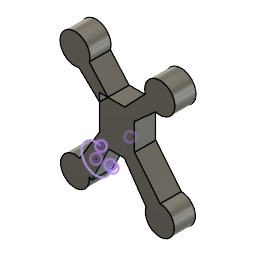
drona (Autodesk Fusion 360 design; units mm, degrees)
part number: 2026-07-06-18-59-21-464
Autodesk Fusion 360 part; units mm, degrees
sketch "Sketch1" plane through (0, 0, 0) normal (0, 0, 1) x (1, 0, 0)
  line L0 (-84.5803, 129.3728) -> (80, 129.3728)
  line L1 (80, 129.3728) -> (80, -80)
  line L2 (80, -80) -> (-84.5803, -80)
  line L3 (-84.5803, -80) -> (-84.5803, 129.3728)
  line L4 (-150, 250) -> (-200, 200)
  line L5 (-200, 200) -> (-84.5803, 90.0801)
  line L6 (-44.3949, 129.3728) -> (-84.5803, 90.0801)
  line L7 (-150, 250) -> (-44.3949, 129.3728)
  constraint horizontal L0
  constraint vertical L1
  constraint horizontal L2
  constraint vertical L3
  constraint coincident L3 L5.end
  constraint coincident L0 L6.start
sketch "Sketch2" plane through (0, 0, 0) normal (0, 0, 1) x (1, 0, 0)
sketch "Sketch3" plane through (0, 0, 0) normal (0, 0, 1) x (1, 0, 0)
sketch "Sketch4" plane through (0, 0, 0) normal (0, 0, 1) x (1, 0, 0)
  line L0 (36.1891, 130.6348) -> (78.7424, 91.729)
  line L1 (200, 200) -> (78.7424, 91.729)
  line L2 (200, 200) -> (150, 250)
  line L3 (150, 250) -> (36.1891, 130.6348)
sketch "Sketch5" plane through (0, 0, 0) normal (0, 0, 1) x (1, 0, 0)
  line L0 (-82.675, -29.7873) -> (-38.9059, -78.4196)
  line L1 (-38.9059, -78.4196) -> (-120.6501, -247.4815)
  line L2 (-120.6501, -247.4815) -> (-189.9512, -207.3598)
  line L3 (-189.9512, -207.3598) -> (-82.675, -29.7873)
sketch "Sketch6" plane through (0, 0, 0) normal (0, 0, 1) x (1, 0, 0)
  line L0 (31.611, -78.4196) -> (81.4591, -32.2189)
  line L1 (81.4591, -32.2189) -> (213.6971, -196.4176)
  line L2 (213.6971, -196.4176) -> (150, -250)
  line L3 (31.611, -78.4196) -> (150, -250)
sketch "Sketch7" plane through (0, 0, 0) normal (0, 0, 1) x (1, 0, 0)
  circle A0 centre (200, 250) radius 71.2765
  circle A1 centre (200, -250) radius 68.2747
  circle A2 centre (-200, 250) radius 70.7107
  circle A3 centre (-200, -250) radius 67.9593
extrude "Extrude1" add sketch "Sketch1" sketch "Sketch7" sketch "Sketch4" sketch "Sketch6" sketch "Sketch5" along normal blind 100 contours L0 L3 L4 L5 L7 | L0 L1 L2 L3 L6 of sketch 2 of sketch 3 of sketch 4 of sketch 5 makes body 1
surface "SurfacePatch1" add patch along 3 edges at (-64.4876, 129.3728, 0) (-64.4876, 109.7265, 0) (-84.5803, 109.7265, 0) separate body on bodies 1 makes body 2
sketch "Sketch8" plane through (0, 0, 0) normal (0, 0, -1) x (-1, 0, 0)
  line L0 (84.5803, -32.9411) -> (84.5803, 90.0801)
  line L1 (84.5803, 90.0801) -> (44.3949, 129.3728)
  line L2 (44.3949, 129.3728) -> (-37.5695, 129.3728)
  line L3 (-37.5695, 129.3728) -> (-36.1891, 130.6348)
  line L4 (-36.1891, 130.6348) -> (-131.4346, 230.5286)
  arc A0 (-131.4346, 230.5286) -> (-179.5332, 181.7252) centre (-200, 250) ccw
  line L5 (-179.5332, 181.7252) -> (-80, 92.8519)
  line L6 (-80, 92.8519) -> (-80, -33.5713)
  line L7 (-80, -33.5713) -> (-81.4591, -32.2189)
  line L8 (-81.4591, -32.2189) -> (-201.8857, -181.7514)
  arc A1 (-201.8857, -181.7514) -> (-135.188, -228.533) centre (-200, -250) ccw
  line L9 (-135.188, -228.533) -> (-32.7015, -80)
  line L10 (-32.7015, -80) -> (39.67, -80)
  line L11 (120.6501, -247.4815) -> (132.7078, -240.5007)
  line L12 (177.0641, -186.028) -> (84.5803, -32.9411)
  arc A2 (132.7078, -240.5007) -> (177.0641, -186.028) centre (200, -250) ccw
  arc A3 (132.7078, -240.5007) -> (177.0641, -186.028) centre (200, -250) ccw
  arc A4 (132.7078, -240.5007) -> (177.0641, -186.028) centre (200, -250) ccw
  arc A5 (132.7078, -240.5007) -> (177.0641, -186.028) centre (200, -250) ccw
sketch "Sketch9" plane through (-0.8013, 0.3875, 0) normal (0.900284, -0.435303, 0) x (0, 0, -1)
  line L0 (0, -89.2912) -> (-100, -89.2912)
  line L1 (-100, -89.2912) -> (-100, -275.323)
  line L2 (-100, -275.323) -> (0, -275.323)
  line L3 (0, -275.323) -> (0, -89.2912)
